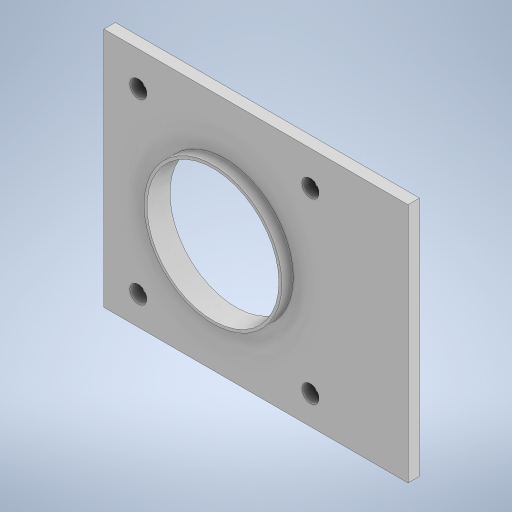
# Autodesk Inventor part: 2
Saved by Autodesk Inventor 2024 (Build 280153000, 153)
## iProperties
Created: 2024-01-05
Part Number: 2
Material: Generic
Document SubType Name: Modeling
Designer: jebes windows
Density: 1 g/cm^3
Appearance: Default
Author: jebes windows
Autodesk Inventor part; units mm, degrees
ref_plane "YZ Plane" through (0, 0, 0) normal (1, 0, 0) x (0, 1, 0)
ref_plane "XZ Plane" through (0, 0, 0) normal (0, 1, 0) x (-1, 0, 0)
ref_plane "XY Plane" through (0, 0, 0) normal (0, 0, 1) x (1, 0, 0)
sketch "Sketch1" plane through (0, 0, 0) normal (0, 1, 0) x (-1, 0, 0)
  line L0 (0, 0) -> (32, 0)
  circle A0 centre (32, 0) radius 12
  line L1 (53, 21) -> (11, 21)
  line L2 (11, 21) -> (11, -21)
  line L3 (11, -21) -> (53, -21)
  line L4 (53, -21) -> (53, 21)
  line L5 (53, 21) -> (11, -21) construction
  line L6 (11, 21) -> (53, -21) construction
  circle A1 centre (47, 15) radius 1.5
  circle A2 centre (47, -16) radius 1.5
  line L7 (32, 0) -> (32, 21)
  circle A3 centre (17, 15) radius 1.5
  circle A4 centre (17, -16) radius 1.5
  line L8 (11, 21) -> (0, 21)
  line L9 (0, 21) -> (0, -21)
  line L10 (0, -21) -> (11, -21)
  dimension "d0" = 32
  dimension "d1" = 24
  dimension "d2" = 42
  dimension "d3" = 42
  dimension "d4" = 3
  dimension "d5" = 3
  dimension "d6" = 31
  dimension "d7" = 15
  dimension "d8" = 15
  dimension "d14" = 11
  constraints: 22 end point, 5 centre point, 3 midpoint, 3 perpendicular, 2 horizontal, 2 parallel, 2 point on line, 2 symmetric about line, 1 coincident, 2 other
  measures "d0" distance of L0.start L0.end
  measures "d1" diameter of A0
  measures "d2" distance of L3.end L2.end
  measures "d3" distance of L2.end L1.end
  measures "d4" diameter of A1
  measures "d5" diameter of A2
  measures "d6" distance of A2.centre A1.centre
  measures "d7" horizontal distance of L0.end A1.centre
  measures "d8" horizontal distance of L0.end A2.centre
  measures "d14" distance between parallel lines of L2 L9
extrude "Extrusion1" add sketch "Sketch1" along normal blind 2 contours L9 L8 L2 L0 | L0 L2 L10 L9 | L2 L1 L7 A0 L0 | L0 A0 L7 L1 L4 L3 L2
sketch "Sketch2" plane through (0, 0, 0) normal (0, -1, 0) x (1, 0, 0)
  line L0 (-53, -21) -> (-53, 21) projected
  circle A0 centre (-17, 15) radius 1.5 projected
  circle A1 centre (-32, 0) radius 12 projected
  circle A2 centre (-17, -16) radius 1.5 projected
  circle A3 centre (-47, 15) radius 1.5 projected
  circle A4 centre (-47, -16) radius 1.5 projected
  circle A5 centre (-32, 0) radius 11.5
  line L1 (0, -21) -> (-53, -21) projected
  line L2 (0, 21) -> (0, -21) projected
  line L3 (-53, 21) -> (0, 21) projected
  point P0 (0, 0)
  dimension "d11" = 23
  constraints: 1 centre point, 1 coincident
  measures "d11" diameter of A5
extrude "Extrusion2" add sketch "Sketch2" along normal mid plane 4 contours A1
body "Solid1"
